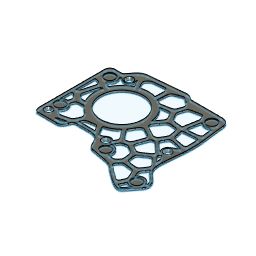
etc (Autodesk Fusion 360 design; units mm, degrees)
Autodesk Fusion 360 part; units mm, degrees
(part 1 of 2)
sketch "스케치4" plane through (0, 0, 0) normal (0, 0, 1) x (1, 0, 0)
  spline S0 degree 3 poles (-87.5156, 61.2226) (-87.8807, 61.1876) (-88.2434, 61.1363) (-88.6019, 61.0697) knots 0 0 0 0 0.033624 0.033624 0.033624 0.033624
  spline S1 degree 3 poles (-22.1324, 49.1151) (-23.6342, 44.0623) (-23.6342, 44.0623) (-31.2248, 41.973) knots -1 -1 -1 -1 0 0 0 0
  spline S2 degree 3 poles (-49.1167, 64.6727) (-49.7355, 64.769) (-50.3835, 64.7862) (-51.0069, 64.7264) knots 0.893415 0.893415 0.893415 0.893415 1 1 1 1
  line L0 (-12.2081, 61.409) -> (-43.1723, 61.409)
  spline S3 degree 3 poles (-47.8588, 64.3608) (-48.2229, 64.4848) (-48.6099, 64.5871) (-49.0168, 64.6565) (-49.0501, 64.6621) (-49.0833, 64.6675) (-49.1167, 64.6727) knots 0.817178 0.817178 0.817178 0.817178 0.887665 0.887665 0.887665 0.893415 0.893415 0.893415 0.893415
  spline S4 degree 3 poles (-11.1719, 61.3885) (-11.5224, 61.4035) (-11.8663, 61.409) (-12.2081, 61.409) knots -0.118565 -0.118565 -0.118565 -0.118565 0 0 0 0
  line L1 (-51.0069, 64.7264) -> (-87.5156, 61.2226)
  spline S5 degree 3 poles (-43.1723, 61.409) (-43.2417, 61.4398) (-43.4397, 61.5515) (-43.7673, 61.7993) (-44.2407, 62.1576) (-44.9274, 62.7887) (-45.9737, 63.4494) (-46.4955, 63.779) (-47.1315, 64.1131) (-47.8588, 64.3608) knots 0.198622 0.198622 0.198622 0.198622 0.393989 0.393989 0.393989 0.676367 0.676367 0.676367 0.817178 0.817178 0.817178 0.817178
  spline S6 degree 5 poles (-47.6334, -11.5321) (-46.8198, -11.5286) (-45.1146, -12.0935) (-42.323, -14.6545) (-38.6965, -20.1619) (-35.0496, -26.8048) (-32.6043, -31.3145) (-31.2223, -33.7861) (-30.7419, -34.6304) knots 0 0 0 0 0 0 0.2 0.4 0.6 0.712041 0.712041 0.712041 0.712041 0.712041 0.712041
  spline S7 degree 3 poles (-88.6019, 61.0697) (-89.7338, 60.8596) (-90.8234, 60.4971) (-91.8131, 60.0127) knots 0.033624 0.033624 0.033624 0.033624 0.139791 0.139791 0.139791 0.139791
  spline S8 degree 5 poles (-37.2011, -46.3427) (-36.5598, -46.2226) (-35.335, -45.8712) (-33.6707, -45.0109) (-31.7946, -43.2974) (-30.1449, -40.5821) (-29.6295, -38.2098) (-29.894, -36.4158) (-30.4037, -35.2247) (-30.7419, -34.6304) knots 0 0 0 0 0 0 0.2 0.4 0.6 0.8 1 1 1 1 1 1
  spline S9 degree 3 poles (-43.5651, 50.8432) (-43.2709, 54.9925) (-43.24, 55.4289) (-38.4365, 57.409) knots -1 -1 -1 -1 -0.105174 -0.105174 -0.105174 -0.105174
  spline S10 degree 3 poles (-31.2248, 41.973) (-38.8154, 39.8838) (-38.8154, 39.8838) (-41.3547, 43.045) knots -1 -1 -1 -1 0 0 0 0
  spline S11 degree 3 poles (-91.8131, 60.0127) (-92.1053, 59.8697) (-92.3888, 59.7162) (-92.662, 59.5527) (-94.5353, 58.4324) (-95.9164, 56.9417) (-97.0355, 55.5438) (-98.3212, 53.9378) (-99.3242, 52.4187) (-100.2323, 51.3674) (-100.9257, 50.5647) (-101.523, 50.0601) (-102.0571, 49.7741) (-102.564, 49.5027) (-103.0402, 49.3595) (-103.8755, 49.3595) knots 0.139791 0.139791 0.139791 0.139791 0.171129 0.171129 0.171129 0.385935 0.385935 0.385935 0.63273 0.63273 0.63273 0.82116 0.82116 0.82116 1 1 1 1
  spline S12 degree 3 poles (-23.2142, -39.5576) (-23.707, -39.1666) (-24.1954, -38.7829) (-24.6907, -38.4039) knots -0.187115 -0.187115 -0.187115 -0.187115 0 0 0 0
  spline S13 degree 5 poles (-69.8015, -15.1659) (-69.6511, -15.1652) (-69.3519, -15.0918) (-68.9072, -14.7655) (-68.3198, -13.9829) (-67.579, -12.799) (-66.9645, -12.0153) (-66.4815, -11.6873) (-66.1477, -11.6124) (-65.9778, -11.6109) knots 0 0 0 0 0 0 0.2 0.4 0.6 0.8 1 1 1 1 1 1
  spline S14 degree 3 poles (-3.0787, -33.4681) (-3.7292, -36.905) (-3.7292, -36.905) (-10.402, -38.9021) knots -1 -1 -1 -1 0 0 0 0
  spline S15 degree 3 poles (-45.6917, -8.9227) (-47.3157, -6.5825) (-47.0773, -5.9887) (-45.5036, -2.07) knots -0.848488 -0.848488 -0.848488 -0.848488 0 0 0 0
  line L2 (-83.8616, 57.5549) -> (-78.0084, 58.1167)
  arc A0 (-105.7469, -3.0986) -> (-112.219, -4.1698) centre (-107.9272, -10.013) ccw
  spline S16 degree 3 poles (-16.1524, -44.9522) (-15.424, -43.497) (-13.8556, -43.0276) (-9.7033, -41.7848) knots -0.622278 -0.622278 -0.622278 -0.622278 0 0 0 0
  spline S17 degree 3 poles (-78.1891, 57.6172) (-78.6044, 56.6643) (-78.6044, 56.6643) (-84.2463, 54.7371) knots -1 -1 -1 -1 0 0 0 0
  line L3 (9.4137, -41.7645) -> (7.7914, -43.8542)
  circle A1 centre (-36.2805, -51.2572) radius 2
  spline S18 degree 5 poles (-115.0132, -25.2175) (-114.9714, -25.4414) (-114.8533, -25.9962) (-114.6076, -26.8618) (-114.129, -27.9562) (-113.3852, -28.7749) (-112.5232, -29.137) (-111.8186, -29.2175) (-111.4337, -29.2175) knots 0.266085 0.266085 0.266085 0.266085 0.266085 0.266085 0.4 0.6 0.8 1 1 1 1 1 1
  spline S19 degree 3 poles (-30.0751, 3.2917) (-27.6799, 1.0482) (-27.6799, 1.0482) (-27.8821, -3.9937) knots -1 -1 -1 -1 0 0 0 0
  line L4 (-88.1757, -15.2433) -> (-69.8015, -15.1659)
  spline S20 degree 3 poles (-27.8821, -3.9937) (-27.9371, -5.3648) (-27.9771, -6.3631) (-28.0903, -7.1499) knots -1 -1 -1 -1 -0.728044 -0.728044 -0.728044 -0.728044
  line L5 (-9.7493, -49.5536) -> (-16.1524, -44.9522)
  arc A2 (-28.3217, -7.223) -> (-42.1967, -11.4316) centre (-35.2805, -9.2572) ccw
  spline S21 degree 3 poles (-45.5036, -2.07) (-43.6489, 2.5486) (-43.6489, 2.5486) (-38.0596, 4.0418) knots -1 -1 -1 -1 0 0 0 0
  spline S22 degree 3 poles (-42.1967, -11.4316) (-42.6424, -10.9815) (-43.0947, -10.5697) (-44.201, -9.6931) (-44.9206, -9.23) (-45.6917, -8.9227) knots -0.627354 -0.627354 -0.627354 -0.627354 -0.451384 -0.451384 -0.202467 -0.202467 -0.202467 -0.202467
  line L6 (-28.0903, -7.1499) -> (-28.3217, -7.223)
  spline S23 degree 3 poles (-26.8144, -35.9324) (-25.7114, -36.2132) (-25.3702, -36.6457) (-23.2142, -39.5576) knots -0.85612 -0.85612 -0.85612 -0.85612 -0.019973 -0.019973 -0.019973 -0.019973
  spline S24 degree 3 poles (-105.8374, -2.7441) (-105.8067, -2.8646) (-105.7765, -2.9827) (-105.7469, -3.0986) knots -1 -1 -1 -1 -0.980817 -0.980817 -0.980817 -0.980817
  line L7 (-115.219, 43.7428) -> (-115.219, -22.9829)
  spline S25 degree 3 poles (-111.5002, 5.2874) (-107.441, 3.5351) (-107.441, 3.5351) (-105.8374, -2.7441) knots -1 -1 -1 -1 0 0 0 0
  circle A3 centre (-93.2805, 47.7428) radius 2
  spline S26 degree 3 poles (-98.5864, -25.2175) (-99.0858, -25.2175) (-99.5687, -25.1457) (-100.4739, -24.8301) (-100.8738, -24.608) (-101.791, -23.9059) (-102.2579, -23.3554) (-102.9147, -22.2151) (-103.2044, -21.522) (-103.3214, -20.6017) knots -1.024159 -1.024159 -1.024159 -1.024159 -0.799804 -0.799804 -0.592815 -0.592815 -0.2783 -0.2783 0 0 0 0
  line L8 (-103.8755, 49.3595) -> (-111.3901, 49.3595)
  spline S27 degree 3 poles (-90.4917, -14.0298) (-90.5282, -14.1068) (-90.5637, -14.186) (-91.1357, -15.526) (-91.4449, -17.2362) (-91.9728, -20.6275) (-92.191, -22.2869) (-92.6487, -23.8888) (-92.7902, -24.279) (-93.0519, -24.729) (-93.1537, -24.8717) (-93.3552, -25.0568) (-93.4432, -25.1175) (-93.6363, -25.1983) (-93.7344, -25.2175) (-93.8366, -25.2175) knots -0.869904 -0.869904 -0.869904 -0.869904 -0.849212 -0.849212 -0.528663 -0.528663 -0.219431 -0.219431 -0.11277 -0.11277 -0.062763 -0.062763 -0.030657 -0.030657 0 0 0 0
  spline S28 degree 3 poles (-101.5367, -13.4371) (-100.1252, -12.3337) (-98.8985, -12.5313) (-94.8066, -13.1905) knots -0.70022 -0.70022 -0.70022 -0.70022 0 0 0 0
  line L9 (-93.8366, -25.2175) -> (-98.5864, -25.2175)
  spline S29 degree 3 poles (1.8289, -26.2176) (-0.4926, -27.3368) (-0.9533, -26.9868) (-5.3426, -23.6518) knots -0.895036 -0.895036 -0.895036 -0.895036 0 0 0 0
  spline S30 degree 3 poles (4.7706, -29.3185) (4.8649, -29.2705) (4.9564, -29.224) (5.0453, -29.179) knots -1 -1 -1 -1 -0.970265 -0.970265 -0.970265 -0.970265
  spline S31 degree 3 poles (-10.4532, -18.7214) (-10.6597, -17.5171) (-10.6597, -17.5171) (-6.5871, -12.3738) knots -1 -1 -1 -1 0 0 0 0
  spline S32 degree 3 poles (-6.5871, -12.3738) (-5.9721, -11.5972) (-5.45, -10.9379) (-4.9994, -10.3783) knots -1 -1 -1 -1 -0.84901 -0.84901 -0.84901 -0.84901
  spline S33 degree 3 poles (-41.3547, 43.045) (-43.8939, 46.2063) (-43.8939, 46.2063) (-43.5651, 50.8432) knots -1 -1 -1 -1 0 0 0 0
  arc A4 (-104.2494, -16.2609) -> (-101.5367, -13.4371) centre (-107.9272, -10.013) ccw
  spline S34 degree 3 poles (-25.0768, 57.409) (-20.6309, 54.1672) (-20.648, 54.1097) (-22.1324, 49.1151) knots -0.988488 -0.988488 -0.988488 -0.988488 0 0 0 0
  spline S35 degree 3 poles (-24.6907, -38.4039) (-25.3077, -37.944) (-26.0181, -37.0907) (-26.8144, -35.9324) knots -3.331847 -3.331847 -3.331847 -3.331847 -2.904031 -2.904031 -2.904031 -2.904031
  spline S36 degree 3 poles (-0.1473, -51.0724) (-1.1352, -52.8336) (-1.6418, -53.7369) (-2.7822, -54.1874) knots -1 -1 -1 -1 -0.512867 -0.512867 -0.512867 -0.512867
  spline S37 degree 5 poles (-115.219, -22.9829) (-115.219, -23.3157) (-115.2036, -23.7612) (-115.1677, -24.2105) (-115.1115, -24.6608) (-115.0338, -25.1071) (-115.0132, -25.2175) knots 0 0 0 0 0 0 0.2 0.266085 0.266085 0.266085 0.266085 0.266085 0.266085
  line L10 (-112.219, -4.1698) -> (-112.219, 5.596)
  spline S38 degree 3 poles (-88.0863, 53.5718) (-87.9901, 53.9092) (-87.876, 54.2389) (-87.5057, 55.1148) (-87.1975, 55.6546) (-86.4619, 56.4994) (-86.0734, 56.816) (-85.0735, 57.3449) (-84.4783, 57.4957) (-83.8616, 57.5549) knots -0.62477 -0.62477 -0.62477 -0.62477 -0.521834 -0.521834 -0.338878 -0.338878 -0.185869 -0.185869 0 0 0 0
  spline S39 degree 3 poles (-9.7033, -41.7848) (-8.3491, -41.3795) (-7.2697, -41.0565) (-6.3888, -40.8311) knots -1 -1 -1 -1 -0.797055 -0.797055 -0.797055 -0.797055
  spline S40 degree 3 poles (-112.219, 5.596) (-111.9938, 5.5005) (-111.755, 5.3974) (-111.5002, 5.2874) knots -0.062774 -0.062774 -0.062774 -0.062774 0 0 0 0
  arc A5 (-103.3214, -20.6017) -> (-105.1465, -17.3371) centre (-108.2815, -21.2322) ccw
  line L11 (5.0453, -29.179) -> (7.3276, -31.2763)
  spline S41 degree 3 poles (-38.0596, 4.0418) (-32.4702, 5.5351) (-32.4702, 5.5351) (-30.0751, 3.2917) knots -1 -1 -1 -1 0 0 0 0
  spline S42 degree 3 poles (-94.8066, -13.1905) (-92.774, -13.518) (-91.4483, -13.7315) (-90.4917, -14.0298) knots -1 -1 -1 -1 -0.652164 -0.652164 -0.652164 -0.652164
  line L12 (-38.4365, 57.409) -> (-25.0768, 57.409)
  line L13 (-111.3901, 49.3595) -> (-111.3896, 49.2322)
  spline S43 degree 3 poles (0.7081, -49.5072) (0.4828, -49.949) (0.197, -50.4586) (-0.1473, -51.0724) knots -0.169767 -0.169767 -0.169767 -0.169767 0 0 0 0
  line L14 (-65.9778, -11.6109) -> (-47.6334, -11.5321)
  spline S44 degree 3 poles (-105.1465, -17.3371) (-104.9004, -17.0095) (-104.6017, -16.6591) (-104.2494, -16.2609) knots -0.198819 -0.198819 -0.198819 -0.198819 -0.065558 -0.065558 -0.065558 -0.065558
  spline S45 degree 3 poles (-78.0084, 58.1167) (-78.0476, 57.9419) (-78.111, 57.7964) (-78.1891, 57.6172) knots -0.188032 -0.188032 -0.188032 -0.188032 0 0 0 0
  spline S46 degree 3 poles (-10.402, -38.9021) (-17.0747, -40.8991) (-17.0747, -40.8991) (-19.7588, -37.2734) knots -1 -1 -1 -1 0 0 0 0
  spline S47 degree 5 poles (-111.3896, 49.2322) (-111.5089, 49.2042) (-111.9526, 49.0837) (-112.6617, 48.7834) (-113.5292, 48.1551) (-114.2294, 47.2936) (-114.6937, 46.396) (-114.9209, 45.739) (-115.0138, 45.385) (-115.0204, 45.3595) knots -0.8715 -0.8715 -0.8715 -0.8715 -0.8715 -0.8715 -0.8 -0.6 -0.4 -0.2 -0.184523 -0.184523 -0.184523 -0.184523 -0.184523 -0.184523
  spline S48 degree 3 poles (-84.2463, 54.7371) (-85.9275, 54.1628) (-87.1078, 53.7596) (-88.0863, 53.5718) knots -1 -1 -1 -1 -0.702015 -0.702015 -0.702015 -0.702015
  spline S49 degree 3 poles (-5.3426, -23.6518) (-10.2467, -19.9257) (-10.2467, -19.9257) (-10.4532, -18.7214) knots -1 -1 -1 -1 0 0 0 0
  spline S50 degree 3 poles (-4.9994, -10.3783) (-4.9161, -11.979) (-4.6694, -13.5688) (-3.8342, -16.955) (-3.1738, -18.792) (-1.0094, -23.1414) (0.5023, -24.947) (1.8289, -26.2176) knots -1.1919 -1.1919 -1.1919 -1.1919 -0.907396 -0.907396 -0.568133 -0.568133 -0.039814 -0.039814 -0.039814 -0.039814
  spline S51 degree 5 poles (-91.6537, -27.4763) (-91.4158, -26.9755) (-90.9684, -25.7324) (-90.4697, -23.3791) (-90.0243, -19.7957) (-89.5419, -16.8166) (-88.963, -15.5318) (-88.458, -15.2445) (-88.1757, -15.2433) knots 0.227373 0.227373 0.227373 0.227373 0.227373 0.227373 0.4 0.6 0.8 1 1 1 1 1 1
  arc A6 (-6.3888, -40.8311) -> (0.7081, -49.5072) centre (0.7195, -42.2572) ccw
  spline S52 degree 3 poles (-2.7822, -54.1874) (-3.3288, -54.0295) (-3.8974, -53.7591) (-6.1168, -52.4472) (-7.836, -50.9285) (-9.7493, -49.5536) knots -0.962437 -0.962437 -0.962437 -0.962437 -0.706834 -0.706834 0 0 0 0
  line L15 (-111.4337, -29.2175) -> (-93.8366, -29.2175)
  spline S53 degree 5 poles (-93.8366, -29.2175) (-93.3333, -29.2175) (-92.8238, -29.0554) (-92.3854, -28.7092) (-92.0112, -28.1995) (-91.6914, -27.5557) (-91.6537, -27.4763) knots 0 0 0 0 0 0 0.2 0.227373 0.227373 0.227373 0.227373 0.227373 0.227373
  spline S54 degree 5 poles (-115.0204, 45.3595) (-115.0985, 45.0555) (-115.1583, 44.7417) (-115.1988, 44.4184) (-115.219, 44.0854) (-115.219, 43.7428) knots -0.184523 -0.184523 -0.184523 -0.184523 -0.184523 -0.184523 0 0 0 0 0 0
  arc A7 (-95.3208, 43.178) -> (-93.6335, 42.7553) centre (-93.2805, 47.7428) ccw
  spline S55 degree 3 poles (-68.386, 46.5035) (-68.6841, 46.9724) (-69.005, 47.4889) (-69.3571, 48.0558) knots -0.088939 -0.088939 -0.088939 -0.088939 0 0 0 0
  spline S56 degree 5 poles (-24.7301, -52.7216) (-24.3219, -52.012) (-23.4703, -50.8243) (-22.5074, -50.0117) (-21.4506, -49.5251) (-20.3273, -49.2981) (-19.7686, -49.2423) knots -1 -1 -1 -1 -1 -1 -0.8 -0.610858 -0.610858 -0.610858 -0.610858 -0.610858 -0.610858
  spline S57 degree 3 poles (-2.9764, 19.7634) (-5.5374, 20.443) (-6.0032, 21.2667) (-7.4048, 23.7445) knots -0.667609 -0.667609 -0.667609 -0.667609 0 0 0 0
  spline S58 degree 3 poles (-3.0851, 15.5791) (-3.0928, 15.4003) (-3.1008, 15.2221) (-3.1092, 15.0445) knots -0.053322 -0.053322 -0.053322 -0.053322 0 0 0 0
  arc A8 (-59.0485, 43.5186) -> (-68.386, 46.5035) centre (-72.1111, 18.7524) ccw
  spline S59 degree 3 poles (-63.3213, 59.0439) (-62.4256, 59.3086) (-61.6175, 59.5473) (-60.8856, 59.7599) knots -1 -1 -1 -1 -0.902272 -0.902272 -0.902272 -0.902272
  spline S60 degree 5 poles (3.4788, -25.0232) (2.8521, -24.4473) (1.7299, -23.2643) (0.4402, -21.3964) (-0.6012, -18.7404) (-1.1515, -15.2068) (-1.2244, -12.2309) (-1.1414, -9.9094) (-1.0291, -8.3186) (-0.9587, -7.5124) knots 0 0 0 0 0 0 0.2 0.4 0.6 0.8 1 1 1 1 1 1
  spline S61 degree 3 poles (-57.1703, 44.0566) (-57.8502, 43.8603) (-58.474, 43.6802) (-59.0485, 43.5186) knots -1 -1 -1 -1 -0.917353 -0.917353 -0.917353 -0.917353
  spline S62 degree 3 poles (-103.2637, 34.0493) (-106.2415, 34.2124) (-108.0595, 34.312) (-109.2526, 34.7932) knots -1 -1 -1 -1 -0.610529 -0.610529 -0.610529 -0.610529
  spline S63 degree 3 poles (0.9499, -34.3676) (1.6004, -30.9307) (1.6004, -30.9307) (4.7706, -29.3185) knots -1 -1 -1 -1 0 0 0 0
  spline S64 degree 3 poles (-7.4048, 23.7445) (-9.5041, 27.4559) (-9.5041, 27.4559) (-9.4719, 27.6838) knots -1 -1 -1 -1 0 0 0 0
  spline S65 degree 5 poles (10.9936, -42.9909) (11.4166, -42.446) (12.1267, -41.3506) (12.6187, -40.1087) (12.8106, -38.8585) (12.7616, -37.6138) (12.6678, -36.9281) (12.6468, -36.7933) knots 0 0 0 0 0 0 0.2 0.4 0.448984 0.448984 0.448984 0.448984 0.448984 0.448984
  spline S66 degree 3 poles (-103.399, 29.5228) (-100.9622, 29.3893) (-99.302, 29.2984) (-98.1062, 29.1569) knots -1 -1 -1 -1 -0.68128 -0.68128 -0.68128 -0.68128
  spline S67 degree 3 poles (-2.4917, 55.0774) (-2.4981, 55.1311) (-2.5051, 55.1848) (-2.5127, 55.2388) (-2.6565, 56.2566) (-3.0528, 57.3507) (-3.6943, 58.2367) (-4.355, 59.1493) (-5.2112, 59.7923) (-5.9935, 60.2051) (-7.0623, 60.7691) (-8.0165, 60.9902) (-8.8787, 61.1421) (-9.6989, 61.2866) (-10.4496, 61.3575) (-11.1719, 61.3885) knots -1 -1 -1 -1 -0.99033 -0.99033 -0.99033 -0.807783 -0.807783 -0.807783 -0.619764 -0.619764 -0.619764 -0.362913 -0.362913 -0.362913 -0.118565 -0.118565 -0.118565 -0.118565
  spline S68 degree 3 poles (0.5272, 9.4975) (0.6134, 10.4843) (0.6899, 11.47) (0.7557, 12.4559) knots 0 0 0 0 0.145343 0.145343 0.145343 0.145343
  spline S69 degree 3 poles (0.7557, 12.4559) (0.9968, 16.0691) (1.0932, 19.6841) (0.9899, 23.3578) (0.9275, 25.5785) (0.7784, 27.8269) (0.5083, 30.0774) knots 0.145343 0.145343 0.145343 0.145343 0.678013 0.678013 0.678013 1 1 1 1
  spline S70 degree 3 poles (-93.9135, 41.463) (-95.6179, 33.6306) (-95.6179, 33.6306) (-103.2637, 34.0493) knots -1 -1 -1 -1 0 0 0 0
  arc A9 (7.7914, -43.8542) -> (0.8296, -35.008) centre (0.7195, -42.2572) ccw
  spline S71 degree 3 poles (-14.4779, -19.6259) (-14.2714, -20.8302) (-14.2714, -20.8302) (-19.3746, -26.3646) knots -1 -1 -1 -1 0 0 0 0
  spline S72 degree 3 poles (-53.1617, 60.5012) (-52.5708, 60.1188) (-51.9989, 59.53) (-51.2209, 58.7288) knots -0.265042 -0.265042 -0.265042 -0.265042 0 0 0 0
  spline S73 degree 3 poles (-51.2209, 58.7288) (-48.2854, 55.7058) (-48.2854, 55.7058) (-48.6142, 51.0689) knots -1 -1 -1 -1 0 0 0 0
  line L16 (0.5083, 30.0774) -> (-2.4917, 55.0774)
  spline S74 degree 3 poles (-30.1183, 38.4692) (-22.5277, 40.5584) (-22.5277, 40.5584) (-18.5096, 34.5094) knots -1 -1 -1 -1 0 0 0 0
  spline S75 degree 5 poles (-0.2805, -55.9596) (-0.2046, -55.9407) (0.3657, -55.7857) (0.9123, -55.5328) (1.4303, -55.169) (1.9162, -54.6841) (2.3137, -54.172) knots -0.230485 -0.230485 -0.230485 -0.230485 -0.230485 -0.230485 -0.2 0 0 0 0 0 0
  spline S76 degree 3 poles (-20.7828, 21.6646) (-13.3015, 25.0361) (-13.3015, 25.0361) (-11.2022, 21.3246) knots -1 -1 -1 -1 0 0 0 0
  spline S77 degree 3 poles (-101.1745, 45.6023) (-100.9042, 45.5924) (-100.6379, 45.5576) (-99.792, 45.3783) (-99.2259, 45.155) (-97.6238, 44.389) (-96.6239, 43.7604) (-95.3208, 43.178) knots -0.778271 -0.778271 -0.778271 -0.778271 -0.668485 -0.668485 -0.428213 -0.428213 0 0 0 0
  spline S78 degree 3 poles (-30.9568, -24.6321) (-33.9875, -18.0769) (-33.9875, -18.0769) (-29.8082, -15.096) knots -1 -1 -1 -1 0 0 0 0
  line L17 (-34.2711, -60.8269) -> (-32.6996, -61.7138)
  spline S79 degree 3 poles (-26.8703, 6.8023) (-29.2654, 9.0457) (-29.2654, 9.0457) (-28.7647, 13.6694) knots -1 -1 -1 -1 0 0 0 0
  spline S80 degree 3 poles (-69.3571, 48.0558) (-73.3167, 54.4304) (-73.3167, 54.4304) (-72.9014, 55.3833) knots -1 -1 -1 -1 0 0 0 0
  spline S81 degree 3 poles (-42.8932, 33.2406) (-43.0361, 30.8678) (-43.0727, 30.2596) (-45.7364, 28.1532) knots -1 -1 -1 -1 -0.256328 -0.256328 -0.256328 -0.256328
  spline S82 degree 3 poles (-30.145, -61.209) (-30.3061, -61.4137) (-30.5056, -61.5849) (-30.959, -61.8413) (-31.2086, -61.9239) (-31.6787, -61.9831) (-31.8934, -61.9757) (-32.3123, -61.8932) (-32.5138, -61.8187) (-32.6996, -61.7138) knots 0 0 0 0 0.078129 0.078129 0.156258 0.156258 0.220292 0.220292 0.284327 0.284327 0.284327 0.284327
  spline S83 degree 3 poles (-28.7647, 13.6694) (-28.264, 18.2931) (-28.264, 18.2931) (-20.7828, 21.6646) knots -1 -1 -1 -1 0 0 0 0
  spline S84 degree 3 poles (-10.9105, 12.3056) (-12.7181, 6.9981) (-12.7181, 6.9981) (-18.5966, 5.7785) knots -1 -1 -1 -1 0 0 0 0
  line L18 (-60.8856, 59.7599) -> (-53.1617, 60.5012)
  spline S85 degree 3 poles (-7.3323, -26.3051) (-2.4282, -30.0311) (-2.4282, -30.0311) (-3.0787, -33.4681) knots -1 -1 -1 -1 0 0 0 0
  spline S86 degree 3 poles (-18.5966, 5.7785) (-24.4752, 4.5588) (-24.4752, 4.5588) (-26.8703, 6.8023) knots -1 -1 -1 -1 0 0 0 0
  spline S87 degree 5 poles (12.6468, -36.7933) (12.5821, -36.378) (12.376, -35.4171) (11.862, -33.93) (11.0855, -32.4986) (10.0538, -31.1599) (9.1623, -30.2461) (8.6809, -29.8037) knots 0.448984 0.448984 0.448984 0.448984 0.448984 0.448984 0.6 0.8 1 1 1 1 1 1
  line L19 (2.3137, -54.172) -> (10.9936, -42.9909)
  line L20 (8.6809, -29.8037) -> (3.4788, -25.0232)
  spline S88 degree 3 poles (-19.7588, -37.2734) (-22.4428, -33.6476) (-22.4428, -33.6476) (-17.3396, -28.1133) knots -1 -1 -1 -1 0 0 0 0
  arc A10 (-37.2011, -46.3427) -> (-40.3959, -54.0969) centre (-36.2805, -51.2572) ccw
  spline S89 degree 3 poles (7.3276, -31.2763) (7.9219, -31.8225) (8.4605, -32.4152) (9.3809, -33.6706) (9.769, -34.3252) (10.419, -35.7835) (10.6664, -36.6148) (10.8123, -38.1563) (10.7624, -38.8456) (10.3491, -40.3495) (9.9389, -41.088) (9.4137, -41.7645) knots -1.188868 -1.188868 -1.188868 -1.188868 -0.947824 -0.947824 -0.722065 -0.722065 -0.467449 -0.467449 -0.256918 -0.256918 0 0 0 0
  spline S90 degree 3 poles (-93.6335, 42.7553) (-93.7205, 42.3496) (-93.8141, 41.9196) (-93.9135, 41.463) knots -0.058301 -0.058301 -0.058301 -0.058301 0 0 0 0
  spline S91 degree 3 poles (-72.9014, 55.3833) (-72.4861, 56.3362) (-72.4861, 56.3362) (-63.3213, 59.0439) knots -1 -1 -1 -1 0 0 0 0
  spline S92 degree 5 poles (-30.145, -61.209) (-30.0481, -61.0859) (-29.7133, -60.654) (-29.142, -59.8796) (-28.3332, -58.7008) (-27.2741, -57.0361) (-26.2833, -55.3895) (-25.5167, -54.083) (-24.9942, -53.1807) (-24.7301, -52.7216) knots -0.440698 -0.440698 -0.440698 -0.440698 -0.440698 -0.440698 -0.4 -0.3 -0.2 -0.1 0 0 0 0 0 0
  line L21 (-3.7687, 32.147) -> (-3.4632, 29.6009)
  line L22 (-0.9587, -7.5124) -> (0.5272, 9.4975)
  spline S93 degree 3 poles (-101.6465, -1.7217) (-103.1549, 4.1852) (-103.2444, 4.5354) (-97.9256, 7.9074) knots -1 -1 -1 -1 -0.05928 -0.05928 -0.05928 -0.05928
  spline S94 degree 3 poles (-17.3396, -28.1133) (-12.2364, -22.579) (-12.2364, -22.579) (-7.3323, -26.3051) knots -1 -1 -1 -1 0 0 0 0
  spline S95 degree 5 poles (-19.7686, -49.2423) (-19.7366, -49.2391) (-19.113, -49.1804) (-17.8677, -49.1971) (-15.9527, -49.5495) (-14.0113, -50.2608) (-12.1522, -51.2231) (-10.9445, -51.9798) (-10.3485, -52.387) knots -0.610858 -0.610858 -0.610858 -0.610858 -0.610858 -0.610858 -0.6 -0.4 -0.2 0 0 0 0 0 0
  spline S96 degree 3 poles (-3.4632, 29.6009) (-3.1696, 27.1539) (-3.0302, 24.749) (-2.9727, 21.4821) (-2.9694, 20.6241) (-2.9764, 19.7634) knots -1.435982 -1.435982 -1.435982 -1.435982 -0.714939 -0.714939 -0.463175 -0.463175 -0.463175 -0.463175
  spline S97 degree 3 poles (-48.6142, 51.0689) (-48.943, 46.4319) (-48.943, 46.4319) (-57.1703, 44.0566) knots -1 -1 -1 -1 0 0 0 0
  spline S98 degree 5 poles (-10.3485, -52.387) (-9.8986, -52.6944) (-8.9626, -53.3039) (-7.45, -54.2026) (-5.3453, -55.2786) (-3.1853, -56.0148) (-1.6489, -56.1792) (-0.7022, -56.0643) (-0.2805, -55.9596) knots -1 -1 -1 -1 -1 -1 -0.8 -0.6 -0.4 -0.230485 -0.230485 -0.230485 -0.230485 -0.230485 -0.230485
  spline S99 degree 3 poles (-19.3746, -26.3646) (-24.4778, -31.8989) (-24.4778, -31.8989) (-26.202, -31.5431) knots -1 -1 -1 -1 0 0 0 0
  spline S100 degree 3 poles (-9.4719, 27.6838) (-9.4424, 27.8926) (-9.44, 27.9101) (-3.7687, 32.147) knots -1 -1 -1 -1 -0.083883 -0.083883 -0.083883 -0.083883
  spline S101 degree 3 poles (-3.1092, 15.0445) (-3.1326, 14.5445) (-3.2139, 14.0559) (-3.5166, 13.1382) (-3.7205, 12.7283) (-4.4759, 11.602) (-5.1588, 10.9702) (-6.4683, 10.0126) (-7.0144, 9.6637) (-7.6135, 9.3047) knots -1.654033 -1.654033 -1.654033 -1.654033 -1.403729 -1.403729 -1.171215 -1.171215 -0.726003 -0.726003 -0.449703 -0.449703 -0.449703 -0.449703
  spline S102 degree 3 poles (-20.1567, -15.2683) (-14.6844, -18.4216) (-14.6844, -18.4216) (-14.4779, -19.6259) knots -1 -1 -1 -1 0 0 0 0
  spline S103 degree 3 poles (0.8296, -35.008) (0.8665, -34.8083) (0.9067, -34.5955) (0.9499, -34.3676) knots -0.066299 -0.066299 -0.066299 -0.066299 0 0 0 0
  arc A11 (-109.2526, 34.7932) -> (-101.1745, 45.6023) centre (-107.3387, 41.786) ccw
  spline S104 degree 3 poles (-11.2022, 21.3246) (-9.1029, 17.6131) (-9.1029, 17.6131) (-10.9105, 12.3056) knots -1 -1 -1 -1 0 0 0 0
  spline S105 degree 3 poles (-26.202, -31.5431) (-27.9261, -31.1873) (-27.9261, -31.1873) (-30.9568, -24.6321) knots -1 -1 -1 -1 0 0 0 0
  spline S106 degree 5 poles (-40.3959, -54.0969) (-40.1942, -54.3892) (-39.7833, -54.9789) (-39.145, -55.8783) (-38.2513, -57.0937) (-37.0564, -58.5624) (-36.0175, -59.6118) (-35.1733, -60.276) (-34.5774, -60.654) (-34.2711, -60.8269) knots 0 0 0 0 0 0 0.2 0.4 0.6 0.8 1 1 1 1 1 1
  spline S107 degree 3 poles (-32.9444, 14.0562) (-33.4452, 9.4326) (-33.4452, 9.4326) (-39.0345, 7.9393) knots -1 -1 -1 -1 0 0 0 0
  spline S108 degree 3 poles (-44.7389, 24.6485) (-40.9, 27.296) (-40.3056, 26.6905) (-36.7311, 23.0484) knots -0.833728 -0.833728 -0.833728 -0.833728 0 0 0 0
  circle A12 centre (-108.2815, -21.2322) radius 2
  spline S109 degree 3 poles (-11.4727, -1.5487) (-9.2136, -3.2291) (-7.6843, -4.2595) (-6.4269, -5.6665) (-6.2573, -5.8754) (-6.1013, -6.093) knots -0.925092 -0.925092 -0.925092 -0.925092 -0.440763 -0.440763 -0.359496 -0.359496 -0.359496 -0.359496
  spline S110 degree 3 poles (-6.1013, -6.093) (-6.4729, -7.1024) (-7.4477, -8.3334) (-9.0637, -10.3742) knots -0.396783 -0.396783 -0.396783 -0.396783 0 0 0 0
  circle A13 centre (-107.9494, -9.9321) radius 5.25
  circle A14 centre (-107.3443, 41.7988) radius 5.25
  spline S111 degree 3 poles (-89.9266, 40.665) (-89.427, 42.9607) (-89.0739, 44.5835) (-88.6822, 45.7792) knots -1 -1 -1 -1 -0.706897 -0.706897 -0.706897 -0.706897
  spline S112 degree 3 poles (-109.3768, 9.6444) (-110.6845, 10.2089) (-111.5709, 10.5915) (-112.219, 11.0639) knots -1 -1 -1 -1 -0.677855 -0.677855 -0.677855 -0.677855
  line L23 (-5.5072, 46.6343) -> (-4.2318, 36.0059)
  spline S113 degree 3 poles (-56.1901, -5.1801) (-56.774, -5.2226) (-57.2904, -5.2602) (-57.7531, -5.2861) knots -1 -1 -1 -1 -0.884294 -0.884294 -0.884294 -0.884294
  spline S114 degree 3 poles (-15.3098, 36.7821) (-19.3279, 42.8311) (-19.3279, 42.8311) (-17.8261, 47.8839) knots -1 -1 -1 -1 0 0 0 0
  spline S115 degree 3 poles (-18.5096, 34.5094) (-14.4916, 28.4604) (-14.4916, 28.4604) (-14.5238, 28.2326) knots -1 -1 -1 -1 0 0 0 0
  line L24 (-70.1544, -12.1673) -> (-84.5419, -12.2279)
  arc A15 (-46.0716, 8.4594) -> (-44.7389, 24.6485) centre (-72.1111, 18.7524) ccw
  circle A16 centre (0.6318, -42.1996) radius 5.25
  spline S116 degree 3 poles (-18.6086, -12.3642) (-24.0809, -9.2109) (-24.0809, -9.2109) (-23.8787, -4.169) knots -1 -1 -1 -1 0 0 0 0
  spline S117 degree 3 poles (-45.2403, 39.5925) (-42.7011, 36.4313) (-42.7011, 36.4313) (-42.8932, 33.2406) knots -1 -1 -1 -1 0 0 0 0
  arc A17 (-57.7531, -5.2861) -> (-48.174, 4.226) centre (-72.1111, 18.7524) ccw
  spline S118 degree 3 poles (-22.0372, 24.6332) (-29.5184, 21.2617) (-29.5184, 21.2617) (-33.8058, 25.6301) knots -1 -1 -1 -1 0 0 0 0
  spline S119 degree 3 poles (-65.0737, -8.3488) (-65.0636, -8.4342) (-65.057, -8.5201) (-65.0539, -8.6069) knots -0.503401 -0.503401 -0.503401 -0.503401 -0.471115 -0.471115 -0.471115 -0.471115
  spline S120 degree 3 poles (-17.798, 2.0925) (-15.9006, 2.4862) (-14.6156, 2.7528) (-13.6289, 2.7897) knots -1 -1 -1 -1 -0.677225 -0.677225 -0.677225 -0.677225
  spline S121 degree 3 poles (-17.8261, 47.8839) (-17.4899, 49.0151) (-17.229, 49.893) (-16.9859, 50.5878) knots -1 -1 -1 -1 -0.77613 -0.77613 -0.77613 -0.77613
  spline S122 degree 3 poles (-23.8787, -4.169) (-23.6765, 0.8729) (-23.6765, 0.8729) (-17.798, 2.0925) knots -1 -1 -1 -1 0 0 0 0
  spline S123 degree 3 poles (-29.8082, -15.096) (-25.6289, -12.115) (-25.6289, -12.115) (-20.1567, -15.2683) knots -1 -1 -1 -1 0 0 0 0
  arc A18 (-16.9859, 50.5878) -> (-5.5072, 46.6343) centre (-9.9556, 52.3592) ccw
  arc A19 (-45.7364, 28.1532) -> (-54.7689, 40.7353) centre (-72.1111, 18.7524) ccw
  spline S124 degree 3 poles (-37.901, 33.1893) (-37.7089, 36.3799) (-37.7089, 36.3799) (-30.1183, 38.4692) knots -1 -1 -1 -1 0 0 0 0
  line L25 (-112.219, 11.0639) -> (-112.219, 28.5454)
  spline S125 degree 3 poles (-7.6135, 9.3047) (-7.4608, 9.7719) (-7.2842, 10.2905) (-7.0859, 10.8729) knots -0.109742 -0.109742 -0.109742 -0.109742 0 0 0 0
  arc A20 (-97.9256, 7.9074) -> (-85.8537, -5.6432) centre (-72.1111, 18.7524) ccw
  spline S126 degree 3 poles (-14.5238, 28.2326) (-14.5559, 28.0047) (-14.5559, 28.0047) (-22.0372, 24.6332) knots -1 -1 -1 -1 0 0 0 0
  circle A21 centre (-8.2805, 2.7428) radius 2
  line L26 (-65.0539, -8.6069) -> (-65.9907, -8.611)
  spline S127 degree 3 poles (-85.8537, -5.6432) (-88.4482, -9.8688) (-89.0916, -9.7652) (-94.1992, -8.9423) knots -0.874031 -0.874031 -0.874031 -0.874031 0 0 0 0
  spline S128 degree 3 poles (-39.0345, 7.9393) (-42.9493, 6.8934) (-44.1222, 6.5801) (-46.0716, 8.4594) knots -1 -1 -1 -1 -0.299607 -0.299607 -0.299607 -0.299607
  spline S129 degree 3 poles (-82.5803, 50.4246) (-77.1668, 52.2738) (-76.9476, 52.3487) (-73.441, 46.7208) knots -1 -1 -1 -1 -0.040498 -0.040498 -0.040498 -0.040498
  spline S130 degree 3 poles (-65.9907, -8.611) (-66.0895, -8.6227) (-66.1853, -8.6525) (-66.3823, -8.7392) (-66.4845, -8.8011) (-66.7949, -9.0193) (-67.0134, -9.2249) (-67.6839, -9.9307) (-68.1513, -10.5316) (-68.8932, -11.3719) (-69.1853, -11.6757) (-69.6037, -11.9844) (-69.7404, -12.0651) (-69.9661, -12.1467) (-70.0593, -12.1669) (-70.1544, -12.1673) knots -0.435151 -0.435151 -0.435151 -0.435151 -0.409126 -0.409126 -0.378744 -0.378744 -0.309484 -0.309484 -0.163433 -0.163433 -0.072132 -0.072132 -0.028544 -0.028544 0 0 0 0
  spline S131 degree 3 poles (-94.1992, -8.9423) (-100.043, -8.0009) (-100.043, -8.0009) (-101.6465, -1.7217) knots -1 -1 -1 -1 0 0 0 0
  spline S132 degree 3 poles (-112.219, 28.5454) (-110.6844, 29.9217) (-109.3848, 29.8506) (-103.399, 29.5228) knots -0.782877 -0.782877 -0.782877 -0.782877 0 0 0 0
  arc A22 (-13.6289, 2.7897) -> (-11.4727, -1.5487) centre (-8.2805, 2.7428) ccw
  line L27 (-90.0093, 40.285) -> (-89.9266, 40.665)
  circle A23 centre (-35.2787, -9.2468) radius 5.25
  spline S133 degree 3 poles (-33.8058, 25.6301) (-38.0931, 29.9986) (-38.0931, 29.9986) (-37.901, 33.1893) knots -1 -1 -1 -1 0 0 0 0
  arc A24 (-98.1062, 29.1569) -> (-99.2168, 11.7323) centre (-72.1111, 18.7524) ccw
  spline S134 degree 3 poles (-36.7311, 23.0484) (-32.4437, 18.6799) (-32.4437, 18.6799) (-32.9444, 14.0562) knots -1 -1 -1 -1 0 0 0 0
  spline S135 degree 3 poles (-88.4754, 46.3602) (-87.5562, 48.7249) (-86.2837, 49.1595) (-82.5803, 50.4246) knots -0.656417 -0.656417 -0.656417 -0.656417 0 0 0 0
  spline S136 degree 3 poles (-84.5419, -12.2279) (-84.6605, -11.0349) (-84.0694, -9.7959) (-82.568, -7.2217) knots -0.608964 -0.608964 -0.608964 -0.608964 -0.105916 -0.105916 -0.105916 -0.105916
  circle A25 centre (-9.9866, 52.3863) radius 5.25
  spline S137 degree 3 poles (-48.174, 4.226) (-47.9828, 3.0578) (-48.4429, 1.9121) (-49.2889, -0.1946) knots -0.456133 -0.456133 -0.456133 -0.456133 0 0 0 0
  circle A26 centre (-72.1111, 18.7524) radius 22
  arc A27 (-73.441, 46.7208) -> (-90.0093, 40.285) centre (-72.1111, 18.7524) ccw
  spline S138 degree 3 poles (-99.2168, 11.7323) (-105.3185, 7.8925) (-105.3809, 7.9194) (-109.3768, 9.6444) knots -0.984405 -0.984405 -0.984405 -0.984405 0 0 0 0
  spline S139 degree 3 poles (-54.7689, 40.7353) (-47.7725, 42.7449) (-47.6453, 42.5866) (-45.2403, 39.5925) knots -0.947112 -0.947112 -0.947112 -0.947112 0 0 0 0
  spline S140 degree 3 poles (-49.2889, -0.1946) (-51.1435, -4.8131) (-51.1435, -4.8131) (-56.1901, -5.1801) knots -1 -1 -1 -1 0 0 0 0
  arc A28 (-82.568, -7.2217) -> (-65.0737, -8.3488) centre (-72.1111, 18.7524) ccw
  arc A29 (-88.6822, 45.7792) -> (-88.4754, 46.3602) centre (-93.2805, 47.7428) ccw
  spline S141 degree 3 poles (-7.0859, 10.8729) (-5.9027, 14.3469) (-5.494, 15.5471) (-3.0851, 15.5791) knots -1 -1 -1 -1 -0.345457 -0.345457 -0.345457 -0.345457
  spline S142 degree 3 poles (-9.0637, -10.3742) (-13.1363, -15.5174) (-13.1363, -15.5174) (-18.6086, -12.3642) knots -1 -1 -1 -1 0 0 0 0
  spline S143 degree 3 poles (-4.2318, 36.0059) (-11.2926, 30.7344) (-11.35, 30.8207) (-15.3098, 36.7821) knots -0.985519 -0.985519 -0.985519 -0.985519 0 0 0 0
extrude "돌출2" add sketch "스케치4" along normal blind 2 makes body 1
extrude "돌출3" cut sketch "스케치4" along normal blind 2 draft 45 contours A1 | A3 | A12 | A21 bodies 1
extrude "돌출4" add sketch "스케치4" along normal blind 1 contours A13 | A14 | A16 | A23 | A25 bodies 1
move_body "이동1" bodies 1 to x (1, 0, 0) y (0, 1, 0) z (0, 0, 1) at (-10, 0, 0)
sketch "스케치7" plane through (0, 0, 0) normal (0, 0, 1) x (1, 0, 0)
  circle A0 centre (16.95, 54.4) radius 2
  spline S0 degree 5 poles (27.4982, -12.7551) (27.5359, -12.7462) (27.7952, -12.6883) (28.3021, -12.6198) (28.8569, -12.6038) (29.4573, -12.6041) (30.0474, -12.6043) (30.3517, -12.6043) knots 0.782864 0.782864 0.782864 0.782864 0.782864 0.782864 0.8 0.9 1 1 1 1 1 1
  line L0 (-1.2033, -22.5603) -> (18.05, -22.5603)
  spline S1 degree 5 poles (-4.7827, -18.5603) (-4.7409, -18.7842) (-4.6228, -19.339) (-4.3771, -20.2046) (-3.8985, -21.299) (-3.1548, -22.1177) (-2.2927, -22.4798) (-1.5881, -22.5603) (-1.2033, -22.5603) knots 0.266085 0.266085 0.266085 0.266085 0.266085 0.266085 0.4 0.6 0.8 1 1 1 1 1 1
  circle A1 centre (101.95, 9.4) radius 2
  spline S2 degree 5 poles (18.05, -22.5603) (18.6197, -22.5603) (19.683, -22.4682) (21.0497, -22.0537) (22.4435, -21.0005) (23.4585, -19.4011) (24.0399, -18.0739) (24.3898, -17.1731) (24.5764, -16.6839) (24.6182, -16.5743) knots 0 0 0 0 0 0 0.1 0.2 0.3 0.4 0.429237 0.429237 0.429237 0.429237 0.429237 0.429237
  circle A2 centre (59.5529, -12.6043) radius 2
  line L1 (30.3517, -12.6043) -> (42.3117, -12.6043)
  spline S3 degree 3 poles (47.0167, -13.2826) (47.3415, -13.3828) (47.6638, -13.4956) (49.5946, -14.2638) (50.7116, -15.1011) (51.9369, -16.2966) (52.306, -16.7248) (52.6396, -17.1685) knots 0.443379 0.443379 0.443379 0.443379 0.534328 0.534328 0.996078 0.996078 1.233253 1.233253 1.233253 1.233253
  spline S4 degree 3 poles (99.882, -45.7298) (101.401, -46.7677) (103.2751, -47.843) (105.8087, -48.886) (106.7014, -49.1848) (107.9736, -49.4038) (108.3756, -49.4439) (109.1724, -49.4404) (109.5654, -49.3979) (109.95, -49.3024) knots 0 0 0 0 0.551913 0.551913 0.815493 0.815493 0.933989 0.933989 1.051154 1.051154 1.051154 1.051154
  spline S5 degree 3 poles (81.6893, -32.1988) (82.3358, -32.4948) (82.9451, -32.873) (84.261, -33.8775) (84.9178, -34.4487) (85.4719, -34.9587) knots 0 0 0 0 0.213325 0.213325 0.400014 0.400014 0.400014 0.400014
  spline S6 degree 5 poles (55.7032, -22.9416) (55.9218, -23.3887) (56.3927, -24.3049) (57.1768, -25.6048) (58.1456, -26.6634) (59.403, -27.3615) (60.4176, -27.6533) (60.9629, -27.7524) knots -0.291341 -0.291341 -0.291341 -0.291341 -0.291341 -0.291341 -0.2 -0.1 0 0 0 0 0 0
  spline S7 degree 3 poles (24.6182, -16.5743) (24.7303, -16.2801) (24.8394, -15.9924) (25.2368, -14.9892) (25.5212, -14.355) (26.1106, -13.5334) (26.3681, -13.2795) (26.9285, -12.9294) (27.2044, -12.8248) (27.4982, -12.7551) knots 0.968464 0.968464 0.968464 0.968464 1.067422 1.067422 1.328044 1.328044 1.501722 1.501722 1.649448 1.649448 1.649448 1.649448
  circle A3 centre (1.949, -14.575) radius 2
  line L2 (60.9629, -27.7524) -> (76.5725, -30.5889)
  spline S8 degree 5 poles (52.6396, -17.1685) (52.7376, -17.2989) (53.1421, -17.8559) (53.8008, -18.9026) (54.395, -20.0885) (54.941, -21.3176) (55.4231, -22.3663) (55.6824, -22.8993) (55.7032, -22.9416) knots -0.531228 -0.531228 -0.531228 -0.531228 -0.531228 -0.531228 -0.5 -0.4 -0.3 -0.291341 -0.291341 -0.291341 -0.291341 -0.291341 -0.291341
  spline S9 degree 3 poles (80.6659, -31.7608) (81.0101, -31.8979) (81.3509, -32.0439) (81.6893, -32.1988) knots 0.427858 0.427858 0.427858 0.427858 0.539492 0.539492 0.539492 0.539492
  spline S10 degree 5 poles (42.3117, -12.6043) (42.8016, -12.6043) (43.7468, -12.6378) (44.6974, -12.7357) (45.6456, -12.9024) (46.5759, -13.1466) (47.0167, -13.2826) knots -1 -1 -1 -1 -1 -1 -0.9 -0.807608 -0.807608 -0.807608 -0.807608 -0.807608 -0.807608
  spline S11 degree 3 poles (76.5725, -30.5889) (77.457, -30.7496) (78.3238, -30.9621) (79.6842, -31.3903) (80.1783, -31.5666) (80.6659, -31.7608) knots -0.539486 -0.539486 -0.539486 -0.539486 -0.269781 -0.269781 -0.111632 -0.111632 -0.111632 -0.111632
  spline S12 degree 3 poles (85.6942, -35.1621) (87.4202, -36.731) (89.3169, -38.2256) (91.1706, -39.6032) knots -1.270613 -1.270613 -1.270613 -1.270613 -0.762618 -0.762618 -0.762618 -0.762618
  spline S13 degree 3 poles (91.1706, -39.6032) (91.5872, -39.9128) (92.0116, -40.2239) (94.7891, -42.2377) (98.0174, -44.4559) (99.882, -45.7298) knots 0.697013 0.697013 0.697013 0.697013 0.835856 0.835856 1.5894 1.5894 1.5894 1.5894
  spline S14 degree 3 poles (121.224, -36.3337) (121.5809, -35.8739) (121.8988, -35.3873) (122.2403, -34.7157) (122.3127, -34.5613) (122.3797, -34.4049) knots -0.502017 -0.502017 -0.502017 -0.502017 -0.379562 -0.379562 -0.343548 -0.343548 -0.343548 -0.343548
  line L3 (112.5442, -47.5148) -> (121.224, -36.3337)
  spline S15 degree 3 poles (109.95, -49.3024) (110.2722, -49.2224) (110.5773, -49.1081) (110.8671, -48.9594) knots 0 0 0 0 0.099596 0.099596 0.099596 0.099596
  spline S16 degree 3 poles (110.8671, -48.9594) (111.0492, -48.8658) (111.2253, -48.7587) (111.8357, -48.3262) (112.214, -47.9402) (112.5442, -47.5148) knots -0.224127 -0.224127 -0.224127 -0.224127 -0.161554 -0.161554 0 0 0 0
  spline S17 degree 3 poles (85.4719, -34.9587) (85.5456, -35.0266) (85.6197, -35.0944) (85.6942, -35.1621) knots 0 0 0 0 0.030071 0.030071 0.030071 0.030071
  line L4 (122.8773, -30.1361) -> (122.8728, -30.1075)
  line L5 (118.9114, -23.1465) -> (113.7092, -18.366)
  spline S18 degree 5 poles (109.1217, -3.0369) (109.1429, -2.607) (109.1687, -2.1739) (109.1987, -1.7376) (109.2331, -1.298) (109.2718, -0.8551) knots 0.890147 0.890147 0.890147 0.890147 0.890147 0.890147 1 1 1 1 1 1
  spline S19 degree 3 poles (110.8227, -14.6294) (110.7389, -14.4658) (110.6581, -14.2994) (109.9567, -12.7701) (109.5529, -11.2716) (109.3181, -9.5719) knots 0.485824 0.485824 0.485824 0.485824 0.541606 0.541606 0.989719 0.989719 0.989719 0.989719
  spline S20 degree 5 poles (109.3181, -9.5719) (109.2887, -9.3598) (109.1715, -8.4302) (109.0735, -7.1556) (109.0401, -5.852) (109.0577, -4.5184) (109.1042, -3.3897) (109.1217, -3.0369) knots 0.540556 0.540556 0.540556 0.540556 0.540556 0.540556 0.6 0.8 0.890147 0.890147 0.890147 0.890147 0.890147 0.890147
  spline S21 degree 3 poles (122.3797, -34.4049) (122.5124, -34.0959) (122.6252, -33.7769) (122.878, -32.8596) (122.9638, -32.2612) (122.9919, -31.145) (122.9554, -30.6377) (122.8773, -30.1361) knots 0.228659 0.228659 0.228659 0.228659 0.331389 0.331389 0.514168 0.514168 0.666674 0.666674 0.666674 0.666674
  spline S22 degree 5 poles (113.7092, -18.366) (113.0825, -17.7901) (112.3981, -17.0686) (111.8113, -16.3239) (111.3139, -15.5577) (110.8956, -14.7717) (110.8227, -14.6294) knots 0 0 0 0 0 0 0.2 0.243958 0.243958 0.243958 0.243958 0.243958 0.243958
  line L6 (109.2718, -0.8551) -> (110.7577, 16.1547)
  spline S23 degree 3 poles (110.7577, 16.1547) (110.7761, 16.3658) (110.7941, 16.5769) (110.8117, 16.7881) knots 0 0 0 0 0.063565 0.063565 0.063565 0.063565
  spline S24 degree 3 poles (111.1944, 23.2094) (111.2472, 24.7513) (111.2699, 26.2937) (111.2377, 30.7357) (111.098, 33.7175) (110.746, 36.6743) knots 0.411131 0.411131 0.411131 0.411131 0.87567 0.87567 1.743969 1.743969 1.743969 1.743969
  line L7 (110.746, 36.6743) -> (110.7388, 36.7347)
  spline S25 degree 3 poles (99.3501, 68.031) (99.2457, 68.0371) (99.1481, 68.0418) (99.0586, 68.0457) knots 1.161785 1.161785 1.161785 1.161785 1.202656 1.202656 1.202656 1.202656
  line L8 (98.0223, 68.0663) -> (67.0582, 68.0663)
  spline S26 degree 3 poles (107.7388, 61.7347) (107.7324, 61.7883) (107.7254, 61.842) (107.7177, 61.896) (107.574, 62.9138) (107.1777, 64.0079) (106.5362, 64.8939) (105.8755, 65.8065) (105.0193, 66.4495) (104.237, 66.8623) (103.1682, 67.4263) (102.2139, 67.6474) (101.3518, 67.7993) (100.6413, 67.9245) (99.983, 67.9945) (99.3501, 68.031) knots -1 -1 -1 -1 -0.99033 -0.99033 -0.99033 -0.807783 -0.807783 -0.807783 -0.619764 -0.619764 -0.619764 -0.362913 -0.362913 -0.362913 -0.151258 -0.151258 -0.151258 -0.151258
  spline S27 degree 3 poles (110.9862, 19.1131) (111.0772, 20.4772) (111.1476, 21.8416) (111.1944, 23.2094) knots 0.145343 0.145343 0.145343 0.145343 0.346451 0.346451 0.346451 0.346451
  spline S28 degree 3 poles (67.0582, 68.0663) (67.011, 68.0872) (66.9051, 68.1451) (65.7624, 68.9208) (64.4315, 70.3164) (62.3717, 71.018) knots 0 0 0 0 0.015471 0.015471 0.107377 0.107377 0.107377 0.107377
  spline S29 degree 3 poles (110.8117, 16.7881) (110.8761, 17.5634) (110.9345, 18.3382) (110.9862, 19.1131) knots 0.031102 0.031102 0.031102 0.031102 0.145343 0.145343 0.145343 0.145343
  spline S30 degree 5 poles (122.8728, -30.1075) (122.8077, -29.698) (122.6007, -28.743) (122.0866, -27.262) (121.3121, -25.8364) (120.2843, -24.5027) (119.3928, -23.5889) (118.9114, -23.1465) knots 0.451068 0.451068 0.451068 0.451068 0.451068 0.451068 0.6 0.8 1 1 1 1 1 1
  spline S31 degree 3 poles (99.0586, 68.0457) (98.8847, 68.0531) (98.7112, 68.0583) (98.3655, 68.0648) (98.1941, 68.0663) (98.0223, 68.0663) knots 0 0 0 0 0.05221 0.05221 0.103736 0.103736 0.103736 0.103736
  spline S32 degree 3 poles (62.3717, 71.018) (62.1708, 71.0864) (61.9673, 71.1468) (61.5484, 71.2518) (61.3324, 71.2959) (61.1138, 71.3299) knots 0 0 0 0 0.063674 0.063674 0.129539 0.129539 0.129539 0.129539
  line L9 (110.7388, 36.7347) -> (107.7388, 61.7347)
  spline S33 degree 3 poles (60.0967, 71.417) (59.8039, 71.4224) (59.5111, 71.4112) (59.2236, 71.3836) knots 0.950836 0.950836 0.950836 0.950836 1 1 1 1
  spline S34 degree 3 poles (21.6286, 67.727) (20.4967, 67.5168) (19.4071, 67.1543) (18.4173, 66.6699) knots 0.033624 0.033624 0.033624 0.033624 0.139791 0.139791 0.139791 0.139791
  line L10 (59.2236, 71.3836) -> (22.7149, 67.8798)
  spline S35 degree 3 poles (-1.9885, 12.9532) (0.642, 12.8377) (1.0617, 12.391) (2.7264, 10.6194) knots 0.252161 0.252161 0.252161 0.252161 1 1 1 1
  spline S36 degree 5 poles (-0.0048, 56.0167) (-0.2523, 56.0167) (-0.4914, 56.0038) (-0.7222, 55.978) (-0.9446, 55.9397) (-1.1591, 55.8894) knots -1 -1 -1 -1 -1 -1 -0.8715 -0.8715 -0.8715 -0.8715 -0.8715 -0.8715
  line L11 (6.3549, 56.0167) -> (-0.0048, 56.0167)
  spline S37 degree 5 poles (-4.7899, 52.0167) (-4.868, 51.7127) (-4.9278, 51.3989) (-4.9683, 51.0756) (-4.9885, 50.7426) (-4.9885, 50.4) knots -0.184523 -0.184523 -0.184523 -0.184523 -0.184523 -0.184523 0 0 0 0 0 0
  spline S38 degree 3 poles (18.4173, 66.6699) (18.1252, 66.527) (17.8417, 66.3734) (17.5684, 66.2099) (16.8437, 65.7765) (16.1925, 65.2876) (15.6018, 64.7701) knots 0.139791 0.139791 0.139791 0.139791 0.171129 0.171129 0.171129 0.254239 0.254239 0.254239 0.254239
  spline S39 degree 3 poles (8.3151, 56.5115) (8.2674, 56.4831) (8.2201, 56.4564) (8.1734, 56.4313) (7.6665, 56.1599) (7.1903, 56.0167) (6.3549, 56.0167) knots 0.804662 0.804662 0.804662 0.804662 0.82116 0.82116 0.82116 1 1 1 1
  spline S40 degree 3 poles (15.6018, 64.7701) (15.374, 64.5705) (15.1414, 64.3546) (13.4577, 62.6927) (12.2967, 61.0383) (10.4268, 58.5174) (9.5803, 57.4187) (8.5424, 56.6544) (8.4248, 56.5769) (8.3151, 56.5115) knots 0.266025 0.266025 0.266025 0.266025 0.323057 0.323057 0.671545 0.671545 0.913262 0.913262 0.946463 0.946463 0.946463 0.946463
  spline S41 degree 5 poles (-1.1591, 55.8894) (-1.2784, 55.8614) (-1.7221, 55.7409) (-2.4312, 55.4407) (-3.2987, 54.8123) (-3.9989, 53.9508) (-4.4632, 53.0532) (-4.6904, 52.3963) (-4.7834, 52.0422) (-4.7899, 52.0167) knots -0.8715 -0.8715 -0.8715 -0.8715 -0.8715 -0.8715 -0.8 -0.6 -0.4 -0.2 -0.184523 -0.184523 -0.184523 -0.184523 -0.184523 -0.184523
  spline S42 degree 3 poles (22.7149, 67.8798) (22.3498, 67.8448) (21.9871, 67.7935) (21.6286, 67.727) knots 0 0 0 0 0.033624 0.033624 0.033624 0.033624
  spline S43 degree 3 poles (61.1138, 71.3299) (60.8023, 71.3784) (60.4855, 71.4065) (60.1458, 71.416) (60.1213, 71.4165) (60.0967, 71.417) knots 0 0 0 0 0.094556 0.094556 0.101928 0.101928 0.101928 0.101928
  spline S44 degree 5 poles (-4.9885, -16.3257) (-4.9885, -16.6585) (-4.9731, -17.104) (-4.9372, -17.5533) (-4.881, -18.0036) (-4.8033, -18.4498) (-4.7827, -18.5603) knots 0 0 0 0 0 0 0.2 0.266085 0.266085 0.266085 0.266085 0.266085 0.266085
  line L12 (-4.9885, 50.4) -> (-4.9885, -16.3257)
  spline S45 degree 3 poles (65.8094, -13.6223) (66.084, -12.8881) (66.6094, -12.028) (67.3903, -10.7496) knots 0.672742 0.672742 0.672742 0.672742 1 1 1 1
  line L13 (-1.9885, 1.7079) -> (-1.9885, 12.9532)
  spline S46 degree 3 poles (84.6409, -15.6433) (85.2817, -20.6484) (85.2817, -20.6484) (83.0913, -23.092) knots 0 0 0 0 1 1 1 1
  spline S47 degree 3 poles (83.0913, -23.092) (80.9008, -25.5357) (80.9008, -25.5357) (75.2025, -24.5352) knots 0 0 0 0 1 1 1 1
  spline S48 degree 3 poles (2.7264, 10.6194) (4.632, 8.5913) (4.9062, 8.2995) (3.6861, 3.6125) knots 0 0 0 0 0.856103 0.856103 0.856103 0.856103
  arc A4 (108.5242, -39.3424) -> (115.565, -40.362) centre (112.95, -33.6) ccw
  spline S49 degree 3 poles (107.4578, -41.4911) (107.8681, -40.5907) (108.1831, -39.8992) (108.5242, -39.3424) knots 0 0 0 0 0.232053 0.232053 0.232053 0.232053
  spline S50 degree 3 poles (79.5769, -8.0329) (84.0001, -10.6382) (84.0001, -10.6382) (84.6409, -15.6433) knots 0 0 0 0 1 1 1 1
  spline S51 degree 3 poles (75.2025, -24.5352) (74.7061, -24.4481) (74.2529, -24.3685) (73.8377, -24.2929) knots 0 0 0 0 0.087122 0.087122 0.087122 0.087122
  arc A5 (3.6861, 3.6125) -> (-1.9885, 1.7079) centre (2.95, -3.6) ccw
  arc A6 (73.8377, -24.2929) -> (65.8094, -13.6223) centre (67.5657, -20.6564) ccw
  spline S52 degree 3 poles (67.3903, -10.7496) (69.7767, -6.843) (69.7767, -6.843) (72.4652, -6.1353) knots 0 0 0 0 1 1 1 1
  spline S53 degree 3 poles (72.4652, -6.1353) (75.1537, -5.4275) (75.1537, -5.4275) (79.5769, -8.0329) knots 0 0 0 0 1 1 1 1
  spline S54 degree 3 poles (110.9644, -46.2884) (110.821, -46.4731) (110.6655, -46.6506) (110.329, -46.9756) (110.1471, -47.1238) (109.95, -47.2499) knots -0.1404 -0.1404 -0.1404 -0.1404 -0.070191 -0.070191 0 0 0 0
  arc A7 (99.2336, 14.0074) -> (98.4059, 5.3942) centre (101.95, 9.4) ccw
  spline S55 degree 3 poles (108.7867, -47.6683) (105.7899, -45.803) (105.7796, -45.7584) (105.7419, -45.5957) knots 0.274119 0.274119 0.274119 0.274119 1 1 1 1
  spline S56 degree 3 poles (2.7587, 25.8604) (1.0781, 19.6449) (0.6568, 18.0869) (-1.9885, 17.6992) knots 0 0 0 0 0.749325 0.749325 0.749325 0.749325
  line L14 (115.565, -40.362) -> (110.9644, -46.2884)
  spline S57 degree 3 poles (107.4692, -18.9538) (108.2551, -17.7905) (108.8404, -16.9242) (109.3117, -16.2751) knots 0 0 0 0 0.255263 0.255263 0.255263 0.255263
  spline S58 degree 3 poles (3.9157, 35.4326) (5.0014, 34.1551) (5.0014, 34.1551) (2.7587, 25.8604) knots 0 0 0 0 1 1 1 1
  spline S59 degree 3 poles (120.9586, -30.633) (120.5785, -30.7342) (120.1615, -30.8441) (119.7038, -30.964) knots 0.78478 0.78478 0.78478 0.78478 0.86224 0.86224 0.86224 0.86224
  spline S60 degree 3 poles (107.0095, -29.4439) (106.8967, -29.1915) (106.7787, -28.9239) (106.6537, -28.6408) knots 0.944803 0.944803 0.944803 0.944803 1 1 1 1
  spline S61 degree 3 poles (109.95, -47.2499) (109.7899, -47.3524) (109.6217, -47.4392) (109.2665, -47.5762) (109.0837, -47.6249) (108.8591, -47.6594) (108.8229, -47.6642) (108.7867, -47.6683) knots -1.365914 -1.365914 -1.365914 -1.365914 -1.277935 -1.277935 -1.189724 -1.189724 -1.172776 -1.172776 -1.172776 -1.172776
  spline S62 degree 5 poles (117.5581, -24.6191) (117.9434, -24.9732) (118.6624, -25.7024) (119.4532, -26.6928) (120.0807, -27.7421) (120.5317, -28.8302) (120.7314, -29.5049) (120.7933, -29.7506) knots 0 0 0 0 0 0 0.2 0.4 0.513664 0.513664 0.513664 0.513664 0.513664 0.513664
  spline S63 degree 3 poles (73.7684, 44.6578) (71.2146, 49.1385) (71.2146, 49.1385) (72.756, 53.7554) knots 0 0 0 0 1 1 1 1
  spline S64 degree 3 poles (88.6138, -15.1197) (87.973, -10.1146) (87.973, -10.1146) (93.1496, -6.4964) knots 0 0 0 0 1 1 1 1
  spline S65 degree 3 poles (83.9136, 11.9478) (85.6002, 12.4525) (85.6002, 12.4525) (91.1663, 7.384) knots 0 0 0 0 1 1 1 1
  arc A8 (60.7321, 8.897) -> (63.6334, 13.8755) centre (38.1194, 25.4096) ccw
  spline S66 degree 5 poles (56.1134, -8.9752) (55.8504, -9.2244) (55.3083, -9.6793) (54.4464, -10.231) (53.3426, -10.6803) (52.1823, -10.9234) (51.3288, -10.9942) (50.8013, -10.996) (50.6068, -10.9909) knots 0 0 0 0 0 0 0.2 0.4 0.6 0.716306 0.716306 0.716306 0.716306 0.716306 0.716306
  spline S67 degree 3 poles (43.3764, 65.8443) (46.3008, 63.5725) (46.2533, 62.7117) (45.8939, 56.2072) knots 0.132339 0.132339 0.132339 0.132339 1 1 1 1
  spline S68 degree 3 poles (91.1663, 7.384) (96.7325, 2.3155) (96.7325, 2.3155) (96.6317, 1.0977) knots 0 0 0 0 1 1 1 1
  spline S69 degree 3 poles (56.6837, 65.6825) (58.8456, 66.4817) (60.2405, 66.9973) (61.3139, 67.1474) knots 0 0 0 0 0.354804 0.354804 0.354804 0.354804
  spline S70 degree 3 poles (29.7031, 52.1147) (29.299, 52.7952) (28.8528, 53.6118) (28.3173, 54.5916) knots 0.833362 0.833362 0.833362 0.833362 1 1 1 1
  spline S71 degree 3 poles (28.3173, 54.5916) (25.2908, 60.1298) (25.1149, 60.4517) (30.2145, 64.5812) knots 0 0 0 0 0.94188 0.94188 0.94188 0.94188
  spline S72 degree 3 poles (80.7542, 59.6559) (87.211, 60.9394) (87.211, 60.9394) (88.714, 58.2763) knots 0 0 0 0 1 1 1 1
  arc A9 (45.617, 52.3871) -> (29.7031, 52.1147) centre (38.1194, 25.4096) ccw
  spline S73 degree 5 poles (62.4132, 66.5304) (62.461, 66.4971) (62.785, 66.2679) (63.3741, 65.8064) (64.1226, 65.1729) (64.8966, 64.6135) (65.6833, 64.2724) (66.1998, 64.1497) (66.4037, 64.1161) knots -0.634509 -0.634509 -0.634509 -0.634509 -0.634509 -0.634509 -0.6 -0.4 -0.2 -0.074302 -0.074302 -0.074302 -0.074302 -0.074302 -0.074302
  spline S74 degree 3 poles (45.8939, 56.2072) (45.8064, 54.6224) (45.7373, 53.3726) (45.617, 52.3871) knots 0 0 0 0 0.211405 0.211405 0.211405 0.211405
  spline S75 degree 3 poles (63.6334, 13.8755) (67.2734, 18.7504) (67.351, 18.7078) (73.1306, 15.5427) knots 0.013442 0.013442 0.013442 0.013442 1 1 1 1
  line L15 (30.2145, 64.5812) -> (43.3764, 65.8443)
  spline S76 degree 3 poles (81.7545, -4.7511) (77.3313, -2.1458) (77.3313, -2.1458) (79.7791, 4.6487) knots 0 0 0 0 1 1 1 1
  spline S77 degree 3 poles (14.2969, 7.3796) (15.2354, 7.3997) (16.0138, 7.4164) (16.6762, 7.4043) knots 0 0 0 0 0.170653 0.170653 0.170653 0.170653